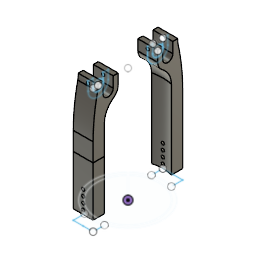
attachment0806 (Autodesk Fusion 360 design; units mm, degrees)
Autodesk Fusion 360 part; units mm, degrees
sketch "Sketch1" plane through (0, 0, 0) normal (0, 0, 1) x (1, 0, 0)
  circle A0 centre (0, 0) radius 35.1
  circle A1 centre (0, 0) radius 31.1
  line L0 (-10, -45.1) -> (-10, -33.6454)
  line L1 (0, -45.1) -> (-10, -45.1)
  line L2 (0, -45.1) -> (10, -45.1)
  line L3 (10, -45.1) -> (10, -33.6454)
  line L4 (10, 45.1) -> (10, 33.6454)
  line L5 (0, 45.1) -> (10, 45.1)
  line L6 (0, 45.1) -> (-10, 45.1)
  line L7 (-10, 45.1) -> (-10, 33.6454)
  dimension "d1" = 70.2
  dimension "d2" = 62.2
  constraint coincident A0.centre A1.centre
  measures "d1" diameter of A0
  measures "d2" diameter of A1
ref_plane "WorkPlane1" through (35, 0, 0) normal (1, 0, 0) x (0, 1, 0)
sketch "Sketch2" plane through (35, 0, 0) normal (1, 0, 0) x (0, 1, 0)
sketch "Sketch3" plane through (0, 0, 0) normal (1, 0, 0) x (0, 1, 0)
  line L0 (0, 0) -> (0, 115)
  line L1 (35.1, 115) -> (35.0791, 115.461)
  line L2 (-35.1, 115) -> (-35.0791, 115.461)
  line L3 (24.9, 115) -> (24.9, 123.7178)
  line L4 (35.1, 115) -> (35.1, 123.7178)
  arc A0 (24.9, 115) -> (35.0791, 115.461) centre (30, 115) ccw
  line L5 (-24.9, 115) -> (-24.9, 123.7178)
  line L6 (-35.1, 115) -> (-35.1, 123.7178)
  arc A1 (-35.0791, 115.461) -> (-24.9, 115) centre (-30, 115) ccw
  line L7 (-19.9, 115) -> (-19.9, 123.7178)
  line L8 (-19.9, 123.7178) -> (-24.9, 123.7178)
  line L9 (-40.1, 115) -> (-40.1, 123.7178)
  line L10 (-35.1, 123.7178) -> (-40.1, 123.7178)
  arc A2 (-40.1, 115) -> (-19.9, 115) centre (-30, 115) ccw
  line L11 (19.9, 115) -> (19.9, 123.7178)
  line L12 (19.9, 123.7178) -> (24.9, 123.7178)
  line L13 (35.1, 123.7178) -> (40.1, 123.7178)
  line L14 (40.1, 115) -> (40.1, 123.7178)
  arc A3 (19.9, 115) -> (40.1, 115) centre (30, 115) ccw
  arc A4 (-35.0791, 115.461) -> (-24.9, 115) centre (-30, 115) ccw
  arc A5 (24.9, 115) -> (35.0791, 115.461) centre (30, 115) ccw
  circle A6 centre (30, 115) radius 5.1
  circle A7 centre (-30, 115) radius 5.1
  dimension "d6" = 115
  dimension "d7" = 30
  dimension "d21" = 10.2
  dimension "d22" = 10.2
  dimension "d53" = 20.2
  dimension "d63" = 10.2
  dimension "d64" = 10.2
  dimension "d89" = 10.2
  dimension "d90" = 10.2
  constraint coincident L0.start origin
  constraint vertical L0
  constraint coincident L1.start A0
  constraint symmetric L0 L1.start L2.start
  constraint concentric A0 A3
  constraint tangent L3 A0
  constraint vertical L3
  constraint tangent L4 A0
  constraint vertical L4
  constraint symmetric L0 L3.start L5.start
  constraint symmetric L0 L4.end L6.end
  constraint symmetric L0 L3.end L5.end
  constraint concentric A1 A4
  constraint concentric A3 A5
  constraint tangent L7 A2
  constraint parallel L5 L7
  constraint perpendicular L5 L8
  constraint tangent L9 A2
  constraint vertical L9
  constraint perpendicular L9 L10
  constraint symmetric L0 L5.end L3.end
  constraint symmetric L0 L6.end L4.end
  constraint symmetric L0 L7.start L11.start
  constraint symmetric L0 L7.end L11.end
  constraint symmetric L0 L9.start L14.start
  constraint symmetric L0 L9.end L13.end
  constraint concentric A0 A6
  constraint concentric A2 A7
  measures "d6" distance of L0.start L0.end
  measures "d7" distance of L0.end A0.centre
  measures "d21" diameter of A1
  measures "d22" diameter of A0
  measures "d53" diameter of A3
  measures "d63" diameter of A4
  measures "d64" diameter of A5
  measures "d89" diameter of A6
  measures "d90" diameter of A7
extrude "Extrude3" add sketch "Sketch1" along normal blind 111 contours A0 L4 L5 L6 L7 | A0 L0 L1 L2 L3 makes body 1 at (1.6894, 35.0593, 74) makes body 2 at (6.7186, -34.451, 74)
extrude "Extrude21" add sketch "Sketch3" along normal blind 10 contours L3 L4 A0 L11 L12 L13 L14 A3 A5 A6 | L5 L6 A1 L7 L8 L9 L10 A2 A4 A7 bodies 2 1
extrude "Extrude22" add sketch "Sketch3" against normal blind 10 contours L3 L4 A0 L11 L12 L13 L14 A3 A5 A6 | L5 L6 A1 L7 L8 L9 L10 A2 A4 A7 bodies 2 1
fillet "Fillet10" radius 20 4 edges at (4.9792, 34.745, 106.084) (-4.9792, 34.745, 106.084) (-4.9792, -34.745, 106.084) (4.9792, -34.745, 106.084) on bodies 1 2
fillet "Fillet11" radius 20 2 edges at (0, 39.2742, 111) (0, -39.2742, 111) on bodies 1 2
fillet "Fillet12" radius 192.5 2 edges at (0, 45.1, 111) (0, -45.1, 111) on bodies 1 2
move_face "OffsetFaces2" offset 2 4 faces at (-3.3333, 21.5667, 123.7178) (-3.3333, 36.7688, 123.7178) (-3.3333, -21.5667, 123.7178) (-3.3333, -36.7688, 123.7178) on bodies 1 2
hole "Hole1" at (-0.0415, -45.1, 121.7881) direction (0, 1, 0) diameter 3.1 depth 110 tip angle 118 bodies 2 1
split "Split1" by plane through (0, 0, 30) normal (0, 0, 1) bodies 1 2 makes body 4 at (7.271, -34.3387, 49.6692) makes body 3 at (7.271, 34.3387, 49.6692)
delete_body "RemoveBody1" bodies 1
delete_body "RemoveBody2" bodies 2
ref_plane "WorkPlane3" through (0, 0, 60) normal (0, 0, 1) x (1, 0, 0)
split "Split2" by plane through (0, 0, 60) normal (0, 0, 1) bodies 4 makes body 5 at (3.3333, -41.5182, 115.3644)
sketch "Sketch4" plane through (0, -45.1, 0) normal (0, -1, 0) x (1, 0, 0)
  line L0 (10, 60) -> (-10, 60)
  line L1 (-10, 60) -> (-10, 30)
  line L2 (-10, 30) -> (10, 30)
  line L3 (10, 30) -> (10, 60)
  circle A0 centre (0, 38) radius 1.5
  circle A1 centre (0, 32) radius 1.5
  circle A2 centre (0, 26) radius 1.55
  circle A3 centre (0, 20) radius 1.55
  circle A4 centre (0, 14) radius 1.55
  line L4 (0, 30.5) -> (0, 30)
  dimension "d104" = 3
  dimension "d105" = 6
  dimension "d106" = 3
  dimension "d115" = 6
  dimension "d116" = 3.1
  dimension "d117" = 6
  dimension "d118" = 3.1
  dimension "d119" = 6
  dimension "d120" = 3.1
  constraint perpendicular L2 L4
  constraint coincident L2 L4.end
  constraint coincident A1 L4.start
  measures "d104" diameter of A0
  measures "d105" distance of A0.centre A1.centre
  measures "d106" diameter of A1
  measures "d115" distance of A1.centre A2.centre
  measures "d116" diameter of A2
  measures "d117" distance of A2.centre A3.centre
  measures "d118" diameter of A3
  measures "d119" distance of A3.centre A4.centre
  measures "d120" diameter of A4
move_face "OffsetFaces3" offset 20 1 faces at (0, -41.7667, 30) on bodies 4
move_face "OffsetFaces4" offset 20 1 faces at (0, 41.7667, 30) on bodies 3
hole "Hole4" at (0, -45.1, 32) at (0, -45.1, 26) at (0, -45.1, 20) at (0, -45.1, 14) direction (0, 1, 0) diameter 3.1 depth 100 tip angle 118 bodies 3 4
